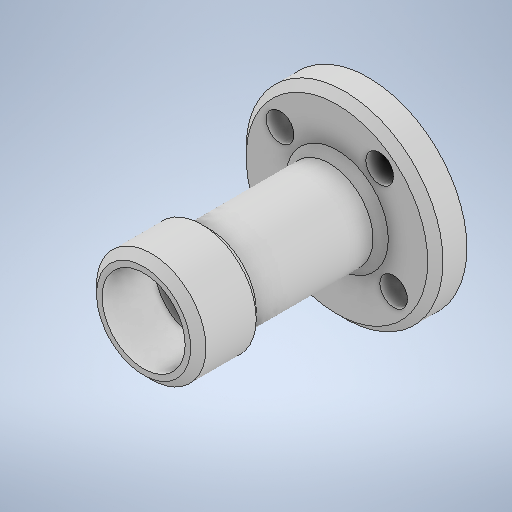
# Autodesk Inventor part: cad@23
Saved by Autodesk Inventor 2025.2 (Build 292293000, 293)
## iProperties
Created: 2025-03-15
Part Number: cad@23
Material: Generic
Document SubType Name: Modeling
Designer: spars
Density: 1 g/cm^3
Appearance: Default
Author: spars
Autodesk Inventor part; units mm, degrees
ref_plane "YZ Plane" through (0, 0, 0) normal (1, 0, 0) x (0, 1, 0)
ref_plane "XZ Plane" through (0, 0, 0) normal (0, 1, 0) x (-1, 0, 0)
ref_plane "XY Plane" through (0, 0, 0) normal (0, 0, 1) x (1, 0, 0)
sketch "Sketch1" plane through (0, 0, 0) normal (0, 0, 1) x (1, 0, 0)
  line L0 (-438.4859, 117.5453) -> (-265.3275, 117.5453) construction
  line L1 (-265.3275, 117.5453) -> (-265.3275, -22.5902) construction
  line L2 (-265.3275, -22.5902) -> (-438.4859, -22.5902) construction
  line L3 (-438.4859, -22.5902) -> (-438.4859, 117.5453) construction
  circle A0 centre (0, 0) radius 45
  dimension "d3" = 90
  constraints: 1 centre point, 1 coincident, 2 other
  measures "d3" diameter of A0
extrude "Extrusion1" add sketch "Sketch1" along normal blind 8 and the other way blind 6.4
sketch "Sketch2" plane through (0, 0, 8) normal (0, 0, 1) x (1, 0, 0)
  circle A0 centre (19.5689, 25.9482) radius 6.35
  circle A1 centre (-25.9482, 19.5689) radius 6.35
  circle A2 centre (-19.5689, -25.9482) radius 6.35
  circle A3 centre (25.9482, -19.5689) radius 6.35
  point P0 (0, 0)
  dimension "d7" = 12.7
  dimension "d8" = 32.5
  dimension "d11" = 360
  constraints: 4 centre point, 9 other
  measures "d7" diameter of A0
  measures "d8" distance of point (0, 0) A0.centre
extrude "Extrusion2" cut sketch "Sketch2" against normal through all
sketch "Sketch3" plane through (0, 0, 8) normal (0, 0, 1) x (1, 0, 0)
  circle A0 centre (0, 0) radius 20
  circle A1 centre (0, 0) radius 15
  dimension "d16" = 40
  dimension "d17" = 30
  constraints: 2 centre point, 2 coincident
  measures "d16" diameter of A0
  measures "d17" diameter of A1
extrude "Extrusion3" add sketch "Sketch3" along normal blind 64.4
sketch "Sketch4" plane through (0, 0, 72.4) normal (0, 0, 1) x (1, 0, 0)
  circle A0 centre (0, 0) radius 25
  circle A1 centre (0, 0) radius 15 projected
  circle A2 centre (0, 0) radius 19
  dimension "d20" = 50
  dimension "d21" = 38
  constraints: 2 centre point, 2 coincident
  measures "d20" diameter of A0
  measures "d21" diameter of A2
extrude "Extrusion4" add sketch "Sketch4" along normal blind 24 and the other way blind 6 contours A0
chamfer "Chamfer1" distance 3.5 angle 45 1 edges at (-20, 0, 8)
chamfer "Chamfer2" distance 3.5 angle 45 1 edges at (-25, 0, 96.4)
chamfer "Chamfer3" distance 3.5 angle 45 1 edges at (-25, 0, 66.4)
chamfer "Chamfer4" distance 3.5 angle 45 1 edges at (-45, 0, 8)
body "Solid1"
